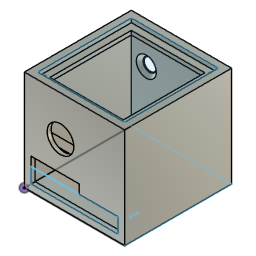
base_robust v1 (Autodesk Fusion 360 design; units mm, degrees)
Autodesk Fusion 360 part; units mm, degrees
sketch "Sketch1" plane through (0, 0, 0) normal (0, 0, 1) x (1, 0, 0)
  line L0 (0, 0) -> (75, 0)
  line L1 (75, 0) -> (75, 80)
  line L2 (75, 80) -> (0, 80)
  line L3 (0, 80) -> (0, 0)
  constraint horizontal L0
  constraint vertical L1
  constraint horizontal L2
  constraint vertical L3
  constraint coincident L0.start L3.end
extrude "Extrude1" add sketch "Sketch1" along normal blind 75
shell "Shell1" thickness 3 removed faces 0 bodies 1
sketch "Sketch2" plane through (0, 0, 0) normal (0, 1, 0) x (1, 0, 0)
  line L0 (5, -5) -> (70, -5)
  line L1 (70, -5) -> (70, -16.2591)
  line L2 (70, -16.2591) -> (5, -16.2591)
  line L3 (5, -16.2591) -> (5, -5)
  constraint horizontal L0
  constraint vertical L1
  constraint horizontal L2
  constraint vertical L3
extrude "Extrude2" cut sketch "Sketch2" along normal blind 5
sketch "Sketch3" plane through (0, 0, 75) normal (0, 0, 1) x (-1, 0, 0)
  line L0 (0, -80) -> (0, 0)
  line L1 (0, 0) -> (-75, 0)
  line L2 (-75, 0) -> (-75, -80)
  line L3 (-75, -80) -> (0, -80)
  line L4 (-70, -5) -> (-5, -5)
  line L5 (-5, -5) -> (-5, -75)
  line L6 (-5, -75) -> (-70, -75)
  line L7 (-70, -75) -> (-70, -5)
  constraint horizontal L4
  constraint vertical L5
  constraint horizontal L6
  constraint vertical L7
extrude "Extrude3" cut sketch "Sketch3" against normal blind 4 contours L4 L5 L6 L7
sketch "Sketch4" plane through (0, 77, 0) normal (0, -1, 0) x (1, 0, 0)
  line L0 (3, 3) -> (72, 3)
  line L1 (72, 3) -> (72, 72)
  line L2 (72, 72) -> (3, 72)
  line L3 (3, 72) -> (3, 3)
sketch "Sketch5" plane through (72, 0, 0) normal (-1, 0, 0) x (0, -1, 0)
  line L0 (-77, 3) -> (-3, 3)
  line L1 (-3, 3) -> (-3, 72)
  line L2 (-3, 72) -> (-77, 72)
  line L3 (-77, 72) -> (-77, 3)
  line L4 (-7, 14) -> (-13, 14)
  line L5 (-13, 14) -> (-13, 13)
  line L6 (-13, 13) -> (-7, 13)
  line L7 (-7, 13) -> (-7, 14)
  constraint horizontal L4
  constraint vertical L5
  constraint horizontal L6
  constraint vertical L7
extrude "Extrude4" add sketch "Sketch5" along normal blind 71 contours L4 L5 L6 L7
sketch "Sketch6" plane through (0, 0, 0) normal (0, -1, 0) x (1, 0, 0)
  line L0 (5, 5) -> (5, 16.2591)
  line L1 (5, 16.2591) -> (70, 16.2591)
  line L2 (70, 16.2591) -> (70, 5)
  line L3 (70, 5) -> (5, 5)
  line L4 (0, 0) -> (75, 0)
  line L5 (75, 0) -> (75, 75)
  line L6 (75, 75) -> (0, 75)
  line L7 (0, 75) -> (0, 0)
  circle A0 centre (27, 45) radius 10
  dimension "d10" = 20
  measures "d10" diameter of A0
extrude "Extrude5" cut sketch "Sketch6" against normal blind 8 contours A0
sketch "Sketch7" plane through (0, 77, 0) normal (0, -1, 0) x (1, 0, 0)
sketch "Sketch8" plane through (0, 77, 0) normal (0, -1, 0) x (1, 0, 0)
  line L0 (75, 72) -> (0, 72)
  line L1 (0, 72) -> (0, 69)
  line L2 (0, 69) -> (75, 69)
  line L3 (75, 69) -> (75, 72)
  constraint horizontal L0
  constraint vertical L1
  constraint horizontal L2
  constraint vertical L3
extrude "Extrude6" add sketch "Sketch8" along normal blind 75
sketch "Sketch9" plane through (0, 0, 75) normal (0, 0, 1) x (-1, 0, 0)
  line L0 (-10, -70) -> (-65, -70)
  line L1 (-65, -70) -> (-65, -9)
  line L2 (-65, -9) -> (-10, -9)
  line L3 (-10, -9) -> (-10, -70)
  constraint horizontal L0
  constraint vertical L1
  constraint horizontal L2
  constraint vertical L3
extrude "Extrude7" cut sketch "Sketch9" against normal blind 12
sketch "Sketch10" plane through (0, 77, 0) normal (0, -1, 0) x (1, 0, 0)
sketch "Sketch11" plane through (0, 0, 75) normal (0, 0, 1) x (-1, 0, 0)
  line L0 (-10, -9) -> (-7, -9)
  line L1 (-7, -9) -> (-7, -7)
  line L2 (-7, -7) -> (-10, -7)
  line L3 (-10, -7) -> (-10, -9)
  constraint horizontal L0
  constraint vertical L1
  constraint horizontal L2
  constraint vertical L3
hole "Hole1" at (7, 7, 75) direction (0, 0, -1) diameter 3 depth 10 tip angle 118
sketch "Sketch12" plane through (0, 0, 75) normal (0, 0, 1) x (-1, 0, 0)
  line L0 (-65, -70) -> (-68, -70)
  line L1 (-68, -70) -> (-68, -72)
  line L2 (-68, -72) -> (-65, -72)
  line L3 (-65, -72) -> (-65, -70)
  constraint horizontal L0
  constraint vertical L1
  constraint horizontal L2
  constraint vertical L3
hole "Hole2" at (68, 72, 75) direction (0, 0, -1) diameter 3 depth 10 tip angle 118
hole "Hole3" at (22.8683, 80, 50.0622) direction (0, -1, 0) diameter 15 depth 10 tip angle 118
sketch "Sketch13" plane through (0, 0, 0) normal (0, 1, 0) x (1, 0, 0)
  line L0 (5, -23) -> (41, -23)
  line L1 (41, -23) -> (41, -5)
  line L2 (41, -5) -> (5, -5)
  line L3 (5, -5) -> (5, -23)
  constraint horizontal L0
  constraint vertical L1
  constraint horizontal L2
  constraint vertical L3
extrude "Extrude8" cut sketch "Sketch13" along normal blind 4
delete_face "DeleteFace1" 1 faces at (49, 7, 13.3333)
sketch "Sketch14" plane through (0, 0, 0) normal (-1, 0, 0) x (0, -1, 0)
  line L0 (-80, 0) -> (0, 0)
  line L1 (0, 0) -> (0, 75)
  line L2 (0, 75) -> (-80, 75)
  line L3 (-80, 75) -> (-80, 0)
  line L4 (-17, 29) -> (-10, 29)
  line L5 (-10, 29) -> (-10, 24)
  line L6 (-10, 24) -> (-17, 24)
  line L7 (-17, 24) -> (-17, 29)
  constraint horizontal L4
  constraint vertical L5
  constraint horizontal L6
  constraint vertical L7
extrude "Extrude9" add sketch "Sketch14" against normal blind 75 contours L4 L5 L6 L7
sketch "Sketch15" plane through (0, 0, 75) normal (0, 0, 1) x (-1, 0, 0)
delete_face "DeleteFace2" 1 faces at (23.6151, 78, 57.525)
hole "Hole4" at (14.2167, 77, 47.1085) direction (0, 1, 0) diameter 10 depth 2.75 tip angle 118 countersink diameter 15 countersink angle 90
